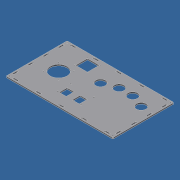
# Autodesk Inventor part: P1704_021
Saved by Autodesk Inventor 2019 (Build 230136000, 136)
## iProperties
Created: 2019-06-21
Part Number: P1704_021
Project: P1704 Manette
Material: .
Description: Couvercle Minotaure
Document SubType Name: Modeling
Designer: Adel.KAHRIMANOVIC
Authority: brut Ø
Density: 0.001 g/cm^3
Appearance: Par défaut
Material number: ---
Author: Adel.KAHRIMANOVIC
Autodesk Inventor part; units mm, degrees
ref_plane "Plan YZ" through (0, 0, 0) normal (1, 0, 0) x (0, 1, 0)
ref_plane "Plan XZ" through (0, 0, 0) normal (0, 1, 0) x (-1, 0, 0)
ref_plane "Plan XY" through (0, 0, 0) normal (0, 0, 1) x (1, 0, 0)
sketch "Esquisse1" plane through (0, 0, 0) normal (0, 0, 1) x (1, 0, 0)
  line L0 (0, 0) -> (315, 0)
  line L1 (315, 0) -> (315, 180)
  line L2 (315, 180) -> (0, 180)
  line L3 (0, 180) -> (0, 0)
  dimension "d0" = 315
  dimension "d1" = 180
  constraints: 8 end point, 2 parallel, 1 horizontal, 1 perpendicular
  measures "d0" distance of L0.start L0.end
  measures "d1" distance of L2.end L0.start
extrude "Extrusion1" add sketch "Esquisse1" along normal blind 4
sketch "Esquisse6" plane through (0, 0, 4) normal (0, 0, 1) x (1, 0, 0)
  line L0 (15, 177) -> (30, 177)
  line L1 (30, 177) -> (30, 172.8)
  line L2 (30, 172.8) -> (15, 172.8)
  line L3 (15, 172.8) -> (15, 177)
  line L4 (157.5, 180) -> (0, 180)
  line L5 (0, 180) -> (0, 0) construction
  line L6 (-223.9576, 90) -> (217.0424, 90) construction
  line L7 (82.5, 177) -> (97.5, 177)
  line L8 (97.5, 177) -> (97.5, 172.8)
  line L9 (97.5, 172.8) -> (82.5, 172.8)
  line L10 (82.5, 172.8) -> (82.5, 177)
  line L11 (150, 177) -> (165, 177)
  line L12 (165, 177) -> (165, 172.8)
  line L13 (165, 172.8) -> (150, 172.8)
  line L14 (150, 172.8) -> (150, 177)
  line L15 (217.5, 177) -> (232.5, 177)
  line L16 (232.5, 177) -> (232.5, 172.8)
  line L17 (232.5, 172.8) -> (217.5, 172.8)
  line L18 (217.5, 172.8) -> (217.5, 177)
  line L19 (285, 177) -> (300, 177)
  line L20 (300, 177) -> (300, 172.8)
  line L21 (300, 172.8) -> (285, 172.8)
  line L22 (285, 172.8) -> (285, 177)
  line L23 (217.5, 7.2) -> (217.5, 3)
  line L24 (232.5, 7.2) -> (217.5, 7.2)
  line L25 (232.5, 3) -> (232.5, 7.2)
  line L26 (285, 7.2) -> (285, 3)
  line L27 (300, 7.2) -> (285, 7.2)
  line L28 (285, 3) -> (300, 3)
  line L29 (300, 3) -> (300, 7.2)
  line L30 (217.5, 3) -> (232.5, 3)
  line L31 (30, 3) -> (30, 7.2)
  line L32 (15, 3) -> (30, 3)
  line L33 (30, 7.2) -> (15, 7.2)
  line L34 (15, 7.2) -> (15, 3)
  line L35 (165, 3) -> (165, 7.2)
  line L36 (150, 3) -> (165, 3)
  line L37 (165, 7.2) -> (150, 7.2)
  line L38 (150, 7.2) -> (150, 3)
  line L39 (97.5, 3) -> (97.5, 7.2)
  line L40 (97.5, 7.2) -> (82.5, 7.2)
  line L41 (82.5, 7.2) -> (82.5, 3)
  line L42 (82.5, 3) -> (97.5, 3)
  line L43 (75.5922, -128.4125) -> (75.5922, 126) construction
  line L44 (0, 180) -> (0, 0) projected
  line L45 (3, 165) -> (7.2, 165)
  line L46 (7.2, 165) -> (7.2, 150)
  line L47 (7.2, 150) -> (3, 150)
  line L48 (3, 150) -> (3, 165)
  line L49 (0, 180) -> (0, -90) construction
  line L50 (157.5, 180) -> (0, 180) construction
  line L51 (157.5, 118.9778) -> (157.5, 83.4509) construction
  line L52 (3, 120) -> (7.2, 120)
  line L53 (7.2, 120) -> (7.2, 105)
  line L54 (7.2, 105) -> (3, 105)
  line L55 (3, 105) -> (3, 120)
  line L56 (3, 75) -> (7.2, 75)
  line L57 (7.2, 75) -> (7.2, 60)
  line L58 (7.2, 60) -> (3, 60)
  line L59 (3, 60) -> (3, 75)
  line L60 (3, 30) -> (7.2, 30)
  line L61 (7.2, 30) -> (7.2, 15)
  line L62 (7.2, 15) -> (3, 15)
  line L63 (3, 15) -> (3, 30)
  line L64 (307.8, 105) -> (312, 105)
  line L65 (307.8, 120) -> (307.8, 105)
  line L66 (312, 105) -> (312, 120)
  line L67 (312, 120) -> (307.8, 120)
  line L68 (307.8, 150) -> (312, 150)
  line L69 (312, 150) -> (312, 165)
  line L70 (307.8, 165) -> (307.8, 150)
  line L71 (312, 165) -> (307.8, 165)
  line L72 (312, 75) -> (307.8, 75)
  line L73 (307.8, 75) -> (307.8, 60)
  line L74 (307.8, 60) -> (312, 60)
  line L75 (312, 30) -> (307.8, 30)
  line L76 (307.8, 30) -> (307.8, 15)
  line L77 (312, 60) -> (312, 75)
  line L78 (312, 15) -> (312, 30)
  line L79 (307.8, 15) -> (312, 15)
  line L80 (315, 180) -> (0, 180) projected
  line L81 (0, 0) -> (315, 180) construction
  line L82 (315, 0) -> (0, 180) construction
  point P0 (157.5, 83.4509)
  point P1 (157.5, 90)
  point P2 (157.5, 90)
  dimension "d107" = 15
  dimension "d108" = 4.2
  dimension "d109" = 3
  dimension "d110" = 15
  dimension "d111" = 67.5
  dimension "d117" = 4.2
  dimension "d118" = 15
  dimension "d119" = 3
  dimension "d120" = 15
  dimension "d121" = 45
  constraints: 156 end point, 32 horizontal alignment, 32 vertical alignment, 18 parallel, 15 collinear, 2 horizontal, 2 midpoint, 2 perpendicular, 2 vertical, 1 coincident, 1 point on line, 12 other
  measures "d107" distance between parallel lines of L1 L3
  measures "d108" distance between parallel lines of L0 L2
  measures "d109" distance between parallel lines of L4 L0
  measures "d110" distance between parallel lines of L3 L5
  measures "d111" distance of L0.start L7.start
  measures "d117" distance between parallel lines of L46 L48
  measures "d118" distance between parallel lines of L47 L45
  measures "d119" distance between parallel lines of L48 L49
  measures "d120" distance between parallel lines of L50 L45
  measures "d121" distance of L45.start L55.end
extrude "Extrusion2" cut sketch "Esquisse6" against normal blind 4
sketch "Esquisse8" plane through (0, 0, 4) normal (0, 0, 1) x (1, 0, 0)
  line L0 (0, 180) -> (0, 0) projected
  line L1 (315, 180) -> (0, 180) projected
  point P0 (5.1, 174.9)
  dimension "d39" = 5.1
  dimension "d40" = 5.1
  measures "d39" distance from line of L0 point (5.1, 174.9)
  measures "d40" distance from line of point (5.1, 174.9) L1
hole "Perçage2" at (5.1, 174.9, 4) direction (0, 0, -1) diameter 3.4 end through all
pattern_linear "Réseau rectangulaire2" count 2 spacing 304.8 along (1, 0, 0) count 2 spacing 169.8 along (0, -1, 0) of "Perçage2"
sketch "Esquisse10" plane through (0, 0, 4) normal (0, 0, 1) x (1, 0, 0)
  circle A0 centre (65, 90) radius 24.75
  line L0 (315, 180) -> (0, 180) projected
  line L1 (-375.2445, 90) -> (140.113, 90) construction
  line L2 (-117.5657, 90) -> (-117.5657, 0) construction
  line L3 (-117.5657, 90) -> (-117.5657, 180) construction
  line L4 (0, 0) -> (315, 0) construction
  line L5 (0, 180) -> (0, 0) construction
  dimension "d64" = 49.5
  dimension "d66" = 65
  constraints: 6 end point, 3 point on line, 2 vertical, 1 centre point, 1 collinear, 1 horizontal, 1 midpoint
  measures "d64" diameter of A0
  measures "d66" distance from line of L5 A0.centre
extrude "Extrusion3" cut sketch "Esquisse10" against normal blind 4
sketch "Esquisse9" plane through (0, 0, 4) normal (0, 0, 1) x (1, 0, 0)
  circle A0 centre (65, 90) radius 24.75 projected
  point P0 (0, 0)
  point P1 (42.5, 112.5)
  dimension "d62" = 22.5
  dimension "d63" = 22.5
  measures "d62" horizontal distance of point (42.5, 112.5) A0.centre
  measures "d63" horizontal distance of A0.centre point (42.5, 112.5)
hole "Perçage3" at (42.5, 112.5, 4) direction (0, 0, -1) diameter 2.9 end through all
pattern_linear "Réseau rectangulaire3" count 2 spacing 45 along (1, 0, 0) count 2 spacing 45 along (0, -1, 0) of "Perçage3"
sketch "Esquisse11" plane through (0, 0, 4) normal (0, 0, 1) x (1, 0, 0)
  line L0 (120, 60) -> (140.7, 60)
  line L1 (140.7, 60) -> (140.7, 36.6)
  line L2 (140.7, 36.6) -> (120, 36.6)
  line L3 (120, 36.6) -> (120, 60)
  line L4 (158.7, 60) -> (179.4, 60)
  line L5 (179.4, 60) -> (179.4, 36.6)
  line L6 (179.4, 36.6) -> (158.7, 36.6)
  line L7 (158.7, 36.6) -> (158.7, 60)
  line L8 (315, 180) -> (0, 180) projected
  line L9 (315, 0) -> (315, 180) projected
  line L10 (0, 180) -> (0, 0) projected
  dimension "d67" = 23.4
  dimension "d68" = 20.7
  dimension "d69" = 18
  dimension "d83" = 120
  dimension "d84" = 120
  constraints: 16 end point, 4 parallel, 3 collinear, 2 horizontal, 2 perpendicular
  measures "d67" distance between parallel lines of L2 L0
  measures "d68" distance of L0.start L0.end
  measures "d69" distance between parallel lines of L7 L1
  measures "d83" distance between parallel lines of L8 L0
  measures "d84" distance between parallel lines of L10 L3
extrude "Extrusion4" cut sketch "Esquisse11" against normal blind 4
sketch "Esquisse12" plane through (0, 0, 4) normal (0, 0, 1) x (1, 0, 0)
  circle A0 centre (277, 121.7188) radius 14
  circle A1 centre (197, 136.7188) radius 14
  circle A2 centre (157, 121.7188) radius 14
  circle A3 centre (237, 136.7188) radius 14
  line L0 (315, 0) -> (315, 180) projected
  line L1 (0, 0) -> (315, 0) projected
  line L2 (315, 180) -> (0, 180) projected
  line L3 (197, 136.7188) -> (215.7332, 136.7188) construction
  line L4 (157, 121.7188) -> (273.4318, 121.7188) construction
  dimension "d77" = 28
  dimension "d97" = 40
  dimension "d98" = 40
  dimension "d99" = 40
  dimension "d100" = 15
  dimension "d101" = 58.2812
  dimension "d102" = 38
  constraints: 4 centre point, 4 end point, 3 equal radius, 2 horizontal, 2 point on line
  measures "d77" diameter of A2
  measures "d97" distance of L3.start A3.centre
  measures "d98" horizontal distance of A3.centre A0.centre
  measures "d99" horizontal distance of L4.start L3.start
  measures "d100" distance between parallel lines of L4 L3
  measures "d101" distance from line of L2 A0.centre
  measures "d102" distance from line of L0 A0.centre
extrude "Extrusion5" cut sketch "Esquisse12" against normal blind 4
sketch "Esquisse13" plane through (0, 0, 4) normal (0, 0, 1) x (1, 0, 0)
  line L0 (120, 36.6) -> (120, 60) projected
  line L1 (120, 60) -> (140.7, 60) projected
  line L2 (140.7, 36.6) -> (120, 36.6) projected
  point P0 (0, 0)
  point P1 (115.5, 37.1)
  dimension "d136" = 4.5
  dimension "d138" = 0.5
  measures "d136" distance from line of point (115.5, 37.1) L0
  measures "d138" distance from line of point (115.5, 37.1) L2
hole "Perçage4" at (115.5, 37.1, 4) direction (0, 0, -1) diameter 3.4 end through all
pattern_linear "Réseau rectangulaire4" count 2 spacing 68.58 along (1, 0, 0) count 2 spacing 38.1 along (0, 1, 0) of "Perçage4"
sketch "Esquisse14" plane through (0, 0, 4) normal (0, 0, 1) x (1, 0, 0)
  line L0 (75, 165) -> (110, 165)
  line L1 (110, 165) -> (110, 130)
  line L2 (110, 130) -> (75, 130)
  line L3 (75, 130) -> (75, 165)
  line L4 (0, 180) -> (0, 0) projected
  line L5 (315, 180) -> (0, 180) projected
  dimension "d139" = 35
  dimension "d140" = 35
  dimension "d160" = 75
  dimension "d161" = 15
  constraints: 8 end point, 2 parallel, 1 horizontal, 1 perpendicular
  measures "d139" distance between parallel lines of L1 L3
  measures "d140" distance between parallel lines of L0 L2
  measures "d160" distance between parallel lines of L4 L3
  measures "d161" distance between parallel lines of L5 L0
extrude "Extrusion6" cut sketch "Esquisse14" against normal blind 10
sketch "Esquisse15" plane through (0, 0, 4) normal (0, 0, 1) x (1, 0, 0)
  line L0 (75, 165) -> (110, 165) projected
  line L1 (75, 130) -> (75, 165) projected
  line L2 (73.5, 166) -> (111.5, 166) construction
  line L3 (111.5, 166) -> (111.5, 129) construction
  line L4 (111.5, 129) -> (73.5, 129) construction
  line L5 (73.5, 129) -> (73.5, 166) construction
  line L6 (75, 130) -> (110, 165) construction
  line L7 (110, 130) -> (75, 165) construction
  line L8 (82.1393, 147.5) -> (102.401, 147.5) construction
  line L9 (92.5, 147.5) -> (92.5, 159.5657) construction
  point P0 (0, 0)
  dimension "d158" = 37
  dimension "d159" = 38
  constraints: 16 end point, 8 point on line, 2 horizontal, 2 parallel, 2 perpendicular, 1 coincident, 1 midpoint, 1 vertical, 2 other
  measures "d158" distance between parallel lines of L4 L2
  measures "d159" distance of L2.start L2.end
hole "Perçage5" at (73.5, 166, 4) at (111.5, 166, 4) at (111.5, 129, 4) at (73.5, 129, 4) direction (0, 0, -1) diameter 2.9 end through all
fillet "Congé1" radius 2 4 edges at (0, 180, 2) (0, 0, 2) (315, 0, 2) (315, 180, 2)
